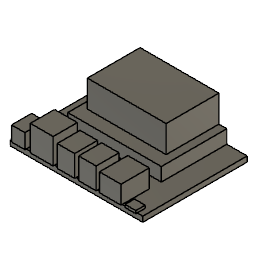
Jetson nano (Autodesk Fusion 360 design; units mm, degrees)
Autodesk Fusion 360 part; units mm, degrees
sketch "Sketch1" plane through (0, 0, 0) normal (0, 0, 1) x (1, 0, 0)
  line L0 (49.35, -38.85) -> (-49.35, -38.85)
  line L1 (-49.35, -38.85) -> (-49.35, 38.85)
  line L2 (-49.35, 38.85) -> (49.35, 38.85)
  line L3 (49.35, 38.85) -> (49.35, -38.85)
  line L4 (49.35, -38.85) -> (-49.35, 38.85) construction
  line L5 (-49.35, -38.85) -> (49.35, 38.85) construction
  dimension "d1" = 98.7
  dimension "d2" = 77.7
  constraint horizontal L0
  constraint perpendicular L0 L1
  constraint parallel L0 L2
  constraint parallel L1 L3
  constraint coincident L4 origin
  constraint coincident L5 origin
  measures "d1" distance of L1.end L2.end
  measures "d2" distance of L0.end L1.end
extrude "Extrude1" add sketch "Sketch1" along normal blind 4
sketch "Sketch2" plane through (0, 0, 4) normal (0, 0, 1) x (-1, 0, 0)
  line L0 (-49.35, -38.85) -> (49.35, -38.85)
  line L1 (49.35, -38.85) -> (49.35, 38.85)
  line L2 (49.35, 38.85) -> (-49.35, 38.85)
  line L3 (-49.35, 38.85) -> (-49.35, -38.85)
  line L4 (35.35, -38.85) -> (-34.25, -38.85)
  line L5 (-34.25, -38.85) -> (-34.25, 9.95)
  line L6 (-34.25, 9.95) -> (35.35, 9.95)
  line L7 (35.35, 9.95) -> (35.35, -38.85)
  dimension "d5" = 69.6
  dimension "d6" = 48.8
  dimension "d7" = 14
  constraint horizontal L4
  constraint vertical L5
  constraint horizontal L6
  constraint vertical L7
  constraint coincident L0 L4.start
  measures "d5" distance of L4.start L4.end
  measures "d6" distance of L4.start L6.end
  measures "d7" distance of L1 L7
extrude "Extrude2" add sketch "Sketch2" along normal blind 10 contours L0 L4 L5 L6 L7
sketch "Sketch3" plane through (0, 0, 14) normal (0, 0, 1) x (-1, 0, 0)
  line L0 (35.35, 9.95) -> (-34.25, 9.95)
  line L1 (-34.25, 9.95) -> (-34.25, -38.85)
  line L2 (-34.25, -38.85) -> (35.35, -38.85)
  line L3 (35.35, -38.85) -> (35.35, 9.95)
  line L4 (30.35, -38.85) -> (-28.35, -38.85)
  line L5 (-28.35, -38.85) -> (-28.35, 0.45)
  line L6 (-28.35, 0.45) -> (30.35, 0.45)
  line L7 (30.35, 0.45) -> (30.35, -38.85)
  dimension "d10" = 39.3
  dimension "d11" = 58.7
  dimension "d12" = 5
  constraint horizontal L4
  constraint vertical L5
  constraint horizontal L6
  constraint vertical L7
  constraint coincident L2 L4.start
  measures "d10" distance of L4.start L6.end
  measures "d11" distance of L4.start L4.end
  measures "d12" distance of L3 L7
extrude "Extrude3" add sketch "Sketch3" along normal blind 20 contours L2 L4 L5 L6 L7
sketch "Sketch4" plane through (0, 0, 4) normal (0, 0, 1) x (-1, 0, 0)
  line L0 (-34.25, -38.85) -> (-34.25, 9.95)
  line L1 (-34.25, 9.95) -> (35.35, 9.95)
  line L2 (35.35, 9.95) -> (35.35, -38.85)
  line L3 (35.35, -38.85) -> (49.35, -38.85)
  line L4 (49.35, -38.85) -> (49.35, 38.85)
  line L5 (49.35, 38.85) -> (-49.35, 38.85)
  line L6 (-49.35, 38.85) -> (-49.35, -38.85)
  line L7 (-49.35, -38.85) -> (-34.25, -38.85)
  line L8 (47.35, 38.85) -> (37.35, 38.85)
  line L9 (37.35, 38.85) -> (37.35, 24.85)
  line L10 (37.35, 24.85) -> (47.35, 24.85)
  line L11 (47.35, 24.85) -> (47.35, 38.85)
  line L12 (33.35, 38.85) -> (16.35, 38.85)
  line L13 (16.35, 38.85) -> (16.35, 21.85)
  line L14 (16.35, 21.85) -> (33.35, 21.85)
  line L15 (33.35, 21.85) -> (33.35, 38.85)
  line L16 (13.35, 38.85) -> (0.35, 38.85)
  line L17 (0.35, 38.85) -> (0.35, 22.85)
  line L18 (0.35, 22.85) -> (13.35, 22.85)
  line L19 (13.35, 22.85) -> (13.35, 38.85)
  line L20 (-2.65, 38.85) -> (-15.65, 38.85)
  line L21 (-15.65, 38.85) -> (-15.65, 22.85)
  line L22 (-15.65, 22.85) -> (-2.65, 22.85)
  line L23 (-2.65, 22.85) -> (-2.65, 38.85)
  line L24 (-18.15, 38.85) -> (-34.15, 38.85)
  line L25 (-34.15, 38.85) -> (-34.15, 18.85)
  line L26 (-34.15, 18.85) -> (-18.15, 18.85)
  line L27 (-18.15, 18.85) -> (-18.15, 38.85)
  line L28 (-37.15, 38.85) -> (-45.15, 38.85)
  line L29 (-45.15, 38.85) -> (-45.15, 32.85)
  line L30 (-45.15, 32.85) -> (-37.15, 32.85)
  line L31 (-37.15, 32.85) -> (-37.15, 38.85)
  dimension "d15" = 10
  dimension "d16" = 14
  dimension "d17" = 17
  dimension "d18" = 17
  dimension "d19" = 2
  dimension "d20" = 4
  dimension "d21" = 13
  dimension "d22" = 16
  dimension "d23" = 13
  dimension "d24" = 16
  dimension "d25" = 3
  dimension "d26" = 3
  dimension "d27" = 16
  dimension "d28" = 20
  dimension "d29" = 2.5
  dimension "d30" = 8
  dimension "d31" = 6
  dimension "d32" = 3
  constraint horizontal L8
  constraint vertical L9
  constraint horizontal L10
  constraint vertical L11
  constraint coincident L5 L8.start
  constraint horizontal L12
  constraint vertical L13
  constraint horizontal L14
  constraint vertical L15
  constraint coincident L5 L12.start
  constraint horizontal L16
  constraint vertical L17
  constraint horizontal L18
  constraint vertical L19
  constraint coincident L5 L16.start
  constraint horizontal L20
  constraint vertical L21
  constraint horizontal L22
  constraint vertical L23
  constraint coincident L5 L20.start
  constraint horizontal L24
  constraint vertical L25
  constraint horizontal L26
  constraint vertical L27
  constraint coincident L5 L24.start
  constraint horizontal L28
  constraint vertical L29
  constraint horizontal L30
  constraint vertical L31
  constraint coincident L5 L28.start
  measures "d15" distance of L8.start L8.end
  measures "d16" distance of L8.start L10.end
  measures "d17" distance of L12.start L12.end
  measures "d18" distance of L12.start L14.end
  measures "d19" distance of L4 L11
  measures "d20" distance of L9 L15
  measures "d21" distance of L16.start L16.end
  measures "d22" distance of L16.start L18.end
  measures "d23" distance of L20.start L20.end
  measures "d24" distance of L20.start L22.end
  measures "d25" distance of L13 L19
  measures "d26" distance of L17 L23
  measures "d27" distance of L24.start L24.end
  measures "d28" distance of L24.start L26.end
  measures "d29" distance of L21 L27
  measures "d30" distance of L28.start L28.end
  measures "d31" distance of L28.start L30.end
  measures "d32" distance of L25 L30.end
extrude "Extrude4" add sketch "Sketch4" along normal blind 11 contours L5 L8 L9 L10 L11
extrude "Extrude5" add sketch "Sketch4" along normal blind 19 contours L5 L12 L13 L14 L15
extrude "Extrude6" add sketch "Sketch4" along normal blind 16 contours L5 L20 L21 L22 L23 | L5 L16 L17 L18 L19
extrude "Extrude7" add sketch "Sketch4" along normal blind 13.5 contours L5 L24 L25 L26 L27
extrude "Extrude8" add sketch "Sketch4" along normal blind 2 contours L5 L28 L29 L30 L31
sketch "Sketch5" plane through (0, -38.85, 0) normal (0, -1, 0) x (1, 0, 0)
  line L0 (-49.35, 0) -> (49.35, 0)
  line L1 (49.35, 0) -> (49.35, 4)
  line L2 (49.35, 4) -> (45.15, 4)
  line L3 (45.15, 4) -> (45.15, 6)
  line L4 (45.15, 6) -> (37.15, 6)
  line L5 (37.15, 6) -> (37.15, 4)
  line L6 (37.15, 4) -> (34.15, 4)
  line L7 (34.15, 4) -> (34.15, 17.5)
  line L8 (34.15, 17.5) -> (18.15, 17.5)
  line L9 (18.15, 17.5) -> (18.15, 4)
  line L10 (18.15, 4) -> (15.65, 4)
  line L11 (15.65, 4) -> (15.65, 20)
  line L12 (15.65, 20) -> (2.65, 20)
  line L13 (2.65, 20) -> (2.65, 4)
  line L14 (2.65, 4) -> (-0.35, 4)
  line L15 (-0.35, 4) -> (-0.35, 20)
  line L16 (-0.35, 20) -> (-13.35, 20)
  line L17 (-13.35, 20) -> (-13.35, 4)
  line L18 (-13.35, 4) -> (-16.35, 4)
  line L19 (-16.35, 4) -> (-16.35, 23)
  line L20 (-16.35, 23) -> (-33.35, 23)
  line L21 (-33.35, 23) -> (-33.35, 4)
  line L22 (-33.35, 4) -> (-37.35, 4)
  line L23 (-37.35, 4) -> (-37.35, 15)
  line L24 (-37.35, 15) -> (-47.35, 15)
  line L25 (-47.35, 15) -> (-47.35, 4)
  line L26 (-47.35, 4) -> (-49.35, 4)
  line L27 (-49.35, 4) -> (-49.35, 0)
  line L28 (-47.35, 4) -> (-37.35, 4)
  line L29 (-37.35, 4) -> (-37.35, 15)
  line L30 (-37.35, 15) -> (-47.35, 15)
  line L31 (-47.35, 15) -> (-47.35, 4)
  line L32 (-33.35, 4) -> (-16.35, 4)
  line L33 (-16.35, 4) -> (-16.35, 23)
  line L34 (-16.35, 23) -> (-33.35, 23)
  line L35 (-33.35, 23) -> (-33.35, 4)
  line L36 (-13.35, 4) -> (-0.35, 4)
  line L37 (-0.35, 4) -> (-0.35, 20)
  line L38 (-0.35, 20) -> (-13.35, 20)
  line L39 (-13.35, 20) -> (-13.35, 4)
  line L40 (2.65, 4) -> (15.65, 4)
  line L41 (15.65, 4) -> (15.65, 20)
  line L42 (15.65, 20) -> (2.65, 20)
  line L43 (2.65, 20) -> (2.65, 4)
  line L44 (18.15, 4) -> (34.15, 4)
  line L45 (34.15, 4) -> (34.15, 17.5)
  line L46 (34.15, 17.5) -> (18.15, 17.5)
  line L47 (18.15, 17.5) -> (18.15, 4)
  line L48 (37.15, 4) -> (45.15, 4)
  line L49 (45.15, 4) -> (45.15, 6)
  line L50 (45.15, 6) -> (37.15, 6)
  line L51 (37.15, 6) -> (37.15, 4)
  constraint horizontal L28
  constraint vertical L29
  constraint horizontal L30
  constraint vertical L31
  constraint coincident L23.end L24.start
  constraint coincident L25.end L26.start
  constraint horizontal L32
  constraint vertical L33
  constraint horizontal L34
  constraint vertical L35
  constraint coincident L19.end L20.start
  constraint coincident L21.end L22.start
  constraint horizontal L36
  constraint vertical L37
  constraint horizontal L38
  constraint vertical L39
  constraint coincident L15.end L16.start
  constraint coincident L17.end L18.start
  constraint horizontal L40
  constraint vertical L41
  constraint horizontal L42
  constraint vertical L43
  constraint coincident L11.end L12.start
  constraint coincident L13.end L14.start
  constraint horizontal L44
  constraint vertical L45
  constraint horizontal L46
  constraint vertical L47
  constraint coincident L7.end L8.start
  constraint coincident L9.end L10.start
  constraint horizontal L48
  constraint vertical L49
  constraint horizontal L50
  constraint vertical L51
  constraint coincident L3.end L4.start
  constraint coincident L5.end L6.start
extrude "Extrude9" add sketch "Sketch5" along normal blind 1 contours L23 L24 L25 L28 L29 L30 L31 | L3 L4 L5 L48 L49 L50 L51 | L19 L20 L21 L32 L33 L34 L35 | L7 L8 L9 L44 L45 L46 L47 | L15 L16 L17 L36 L37 L38 L39 | L11 L12 L13 L40 L41 L42 L43
